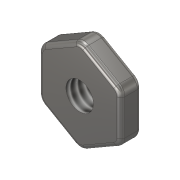
# Autodesk Inventor part: magnet_spacer_nut
Saved by Autodesk Inventor 2019 (Build 230136000, 136)
## iProperties
Created: 2023-10-12
Part Number: magnet_spacer_nut
Material: Steel, Alloy
Document SubType Name: Modeling
Designer: prich
Density: 7.73 g/cm^3
Appearance: Semi-Polished
Mass: 0.192193 g
Surface Area: 0.647024 cm^2
Volume: 0.0248632 cm^3
Author: prich
Autodesk Inventor part; units mm, degrees
ref_plane "YZ Plane" through (0, 0, 0) normal (1, 0, 0) x (0, 1, 0)
ref_plane "XZ Plane" through (0, 0, 0) normal (0, 1, 0) x (-1, 0, 0)
ref_plane "XY Plane" through (0, 0, 0) normal (0, 0, 1) x (1, 0, 0)
sketch "Sketch1" plane through (0, 0, 0) normal (0, 0, 1) x (1, 0, 0)
  line L0 (0, 2.9329) -> (2.54, 1.4665)
  line L1 (2.54, 1.4665) -> (2.54, -1.4665)
  line L2 (2.54, -1.4665) -> (0, -2.9329)
  line L3 (0, -2.9329) -> (-2.54, -1.4665)
  line L4 (-2.54, -1.4665) -> (-2.54, 1.4665)
  line L5 (-2.54, 1.4665) -> (0, 2.9329)
  point P0 (0, 0)
  point P1 (0, 0)
  dimension "d0" = 5.08
  constraints: 12 end point, 1 coincident, 13 other
  measures "d0" distance between parallel lines of L1 L4
extrude "Extrusion1" add sketch "Sketch1" along normal blind 1.27
fillet "Fillet1" radius 0.635 6 edges at (-2.54, -1.4665, 0.635) (0, -2.9329, 0.635) (2.54, -1.4665, 0.635) (-2.54, 1.4665, 0.635) (2.54, 1.4665, 0.635) (0, 2.9329, 0.635)
fillet "Fillet2" radius 0.254 12 edges at (0, 2.8347, 1.27) (-1.27, 2.1997, 1.27) (-2.4549, 1.4174, 1.27) (-2.54, 0, 1.27) (-2.4549, -1.4174, 1.27) (-1.27, -2.1997, 1.27) (0, -2.8347, 1.27) (1.27, -2.1997, 1.27) (2.4549, -1.4174, 1.27) (2.54, 0, 1.27) (2.4549, 1.4174, 1.27) (1.27, 2.1997, 1.27)
fillet "Fillet3" radius 0.254 12 edges at (2.4549, 1.4174, 0) (2.54, 0, 0) (2.4549, -1.4174, 0) (1.27, -2.1997, 0) (0, -2.8347, 0) (-1.27, -2.1997, 0) (-2.4549, -1.4174, 0) (-2.54, 0, 0) (-2.4549, 1.4174, 0) (-1.27, 2.1997, 0) (0, 2.8347, 0) (1.27, 2.1997, 0)
sketch "Sketch2" plane through (0, 0, 1.27) normal (0, 0, 1) x (1, 0, 0)
  point P0 (0, 0)
  point P1 (0, 0)
  constraints: 1 coincident
hole "Hole1" at (0, 0, 1.27) direction (0, 0, -1) diameter 1.7018 depth 6.6294 tip angle 118
body "Solid1"
